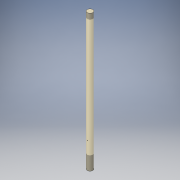
# Autodesk Inventor part: Tongkatttt
Saved by Autodesk Inventor 2019.5 (Build 235369000, 369)
## iProperties
Created: 2022-10-11
Part Number: Tongkatttt
Material: Aluminum 6061-AHC
Document SubType Name: Modeling
Designer: ASUS
Density: 2.7 g/cm^3
Appearance: Aluminum - Dark
Author: ASUS
Autodesk Inventor part; units mm, degrees
ref_plane "YZ Plane" through (0, 0, 0) normal (1, 0, 0) x (0, 1, 0)
ref_plane "XZ Plane" through (0, 0, 0) normal (0, 1, 0) x (-1, 0, 0)
ref_plane "XY Plane" through (0, 0, 0) normal (0, 0, 1) x (1, 0, 0)
sketch "Sketch1" plane through (0, 0, 0) normal (0, 1, 0) x (-1, 0, 0)
  circle A0 centre (0, 0) radius 20
  dimension "d0" = 40
  constraints: 1 centre point, 1 coincident
  measures "d0" diameter of A0
extrude "Extrusion1" add sketch "Sketch1" along normal blind 1000
sketch "Sketch2" plane through (0, 0, 0) normal (0, 0, 1) x (1, 0, 0)
  circle A0 centre (0, 190.0543) radius 1.5
  point P0 (0, 0)
  dimension "d3" = 3
  constraints: 1 centre point
  measures "d3" diameter of A0
extrude "Extrusion2" add sketch "Sketch2" along normal blind 25 and the other way blind 25
sketch "Sketch3" plane through (0, 190.0543, 25) normal (0, 0, 1) x (1, 0, 0)
  point P0 (0, -190.0543)
  point P1 (-0.0211, -0.0123)
hole "Hole1" at (-0.0211, 190.042, 25) direction (0, 0, -1) diameter 4 depth 51
sketch "Sketch4" plane through (0, 0, 0) normal (0, -1, 0) x (1, 0, 0)
  point P0 (0, 0)
  point P1 (0, 0)
  constraints: 1 coincident
hole "Hole2" at (0, 0, 0) direction (0, 1, 0) diameter 29 depth 906
thread "Thread2" size "M40x3" class "6g" standard "ANSI Metric M Profile" length 40
thread "Thread3" size "M40x3" class "6g" standard "ANSI Metric M Profile" length 100
body "Solid1"
